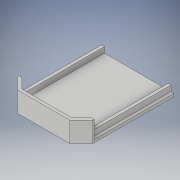
# Autodesk Inventor part: bottom-housing
Saved by Autodesk Inventor 2018 (Build 220112000, 112)
## iProperties
Created: 2019-10-14
Part Number: bottom-housing
Material: Generic
Document SubType Name: Modeling
Designer: jklei
Density: 1 g/cm^3
Appearance: Default
Author: jklei
Autodesk Inventor part; units mm, degrees
ref_plane "YZ Plane" through (0, 0, 0) normal (1, 0, 0) x (0, 1, 0)
ref_plane "XZ Plane" through (0, 0, 0) normal (0, 1, 0) x (-1, 0, 0)
ref_plane "XY Plane" through (0, 0, 0) normal (0, 0, 1) x (1, 0, 0)
sketch "Sketch1" plane through (0, 0, 0) normal (0, 1, 0) x (-1, 0, 0)
  line L0 (0, 0) -> (82.55, 0)
  line L1 (82.55, 0) -> (82.55, -101.6)
  line L2 (82.55, -101.6) -> (0, -101.6)
  line L3 (0, -101.6) -> (0, 0)
  dimension "d0" = 82.55
  dimension "d1" = 101.6
  constraints: 8 end point, 2 parallel, 1 horizontal, 1 perpendicular
  measures "d0" distance of L1.end L2.end
  measures "d1" distance of L0.end L1.end
extrude "Extrusion1" add sketch "Sketch1" along normal blind 3.175
chamfer "Chamfer1" distance 12.7 angle 45 2 edges at (-82.55, 1.5875, 0) (0, 1.5875, 0)
sketch "Sketch9" plane through (0, 3.175, 0) normal (0, 1, 0) x (1, 0, 0)
  line L0 (0, 12.7) -> (-12.7, 0) projected
  line L1 (0, 12.7) -> (0, 101.6) projected
  line L2 (0, 101.6) -> (-82.55, 101.6) projected
  line L3 (-82.55, 101.6) -> (-82.55, 12.7) projected
  line L4 (-69.85, 0) -> (-82.55, 12.7) projected
  line L5 (-69.85, 0) -> (-12.7, 0) projected
  line L6 (-3.175, 14.0151) -> (-14.0151, 3.175)
  line L7 (-14.0151, 3.175) -> (-68.5349, 3.175)
  line L8 (-68.5349, 3.175) -> (-79.375, 14.0151)
  line L9 (-82.55, 101.6) -> (0, 101.6) projected
  line L10 (-79.375, 14.0151) -> (-82.55, 14.0151)
  line L11 (-82.55, 12.7) -> (-82.55, 101.6) projected
  line L12 (-3.175, 14.0151) -> (0, 14.0151)
  point P0 (0, 0)
  point P1 (-3.175, 98.425)
  point P2 (-3.175, 101.6)
  constraints: 10 end point, 3 point on line, 2 horizontal, 2 other
extrude "Extrusion8" add sketch "Sketch9" along normal blind 19.05 contours L0 L5 L4 L3 L10 L8 L7 L6 L12 L1
sketch "Sketch12" plane through (0, 3.175, 0) normal (0, 1, 0) x (1, 0, 0)
  line L0 (0, 101.6) -> (-82.55, 101.6) projected
  line L1 (0, 101.6) -> (-3.175, 101.6)
  line L2 (-14.0151, 3.175) -> (-3.175, 14.0151) projected
  line L3 (-3.175, 101.6) -> (-6.35, 101.6)
  line L4 (-6.35, 101.6) -> (-6.35, 12.7)
  line L5 (-6.35, 12.7) -> (-3.175, 12.7)
  line L6 (-3.175, 12.7) -> (-3.175, 101.6)
  line L7 (-82.55, 101.6) -> (-79.375, 101.6)
  line L8 (-79.375, 101.6) -> (-76.2, 101.6)
  line L9 (-76.2, 101.6) -> (-76.2, 12.7)
  line L10 (-76.2, 12.7) -> (-79.375, 12.7)
  line L11 (-79.375, 12.7) -> (-79.375, 101.6)
  point P0 (0, 0)
  dimension "d34" = 3.175
  dimension "d35" = 3.175
  dimension "d36" = 88.9
  dimension "d37" = 3.175
  dimension "d38" = 3.175
  dimension "d39" = 88.9
  constraints: 20 end point, 4 parallel, 2 horizontal, 2 perpendicular, 2 point on line
  measures "d34" distance of L0.start L1.end
  measures "d35" distance of L5.end L4.end
  measures "d36" distance of L4.end L3.end
  measures "d37" distance of L0.end L7.end
  measures "d38" distance of L9.end L10.end
  measures "d39" distance of L8.end L9.end
extrude "Extrusion10" add sketch "Sketch12" along normal blind 6.35
body "Solid1"
